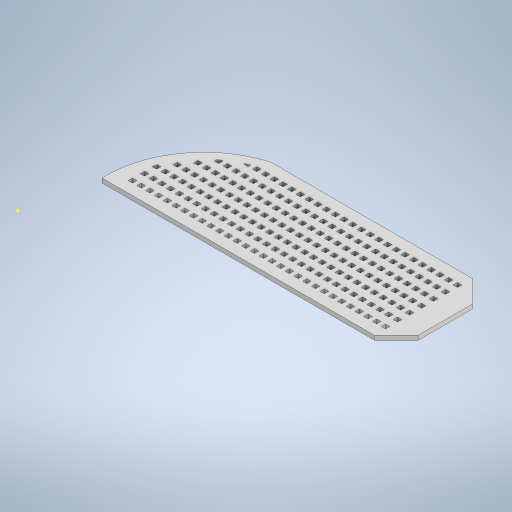
# Autodesk Inventor part: Cover_1
Saved by Autodesk Inventor 2024 (Build 280153000, 153)
## iProperties
Created: 2023-11-10
Part Number: Cover_1
Material: Generic
Document SubType Name: Modeling
Designer: furqa
Density: 1 g/cm^3
Appearance: Default
Author: furqa
Autodesk Inventor part; units mm, degrees
(part 1 of 2)
ref_plane "YZ Plane" through (0, 0, 0) normal (1, 0, 0) x (0, 1, 0)
ref_plane "XZ Plane" through (0, 0, 0) normal (0, 1, 0) x (-1, 0, 0)
ref_plane "XY Plane" through (0, 0, 0) normal (0, 0, 1) x (1, 0, 0)
sketch "Sketch1" plane through (0, 0, 0) normal (0, 1, 0) x (-1, 0, 0)
  line L0 (-38.923, -75.3658) -> (-131.4067, -75.3658)
  line L1 (-131.4067, -34.3658) -> (-8.4067, -34.3658)
  line L2 (-8.4067, -34.3658) -> (-8.4067, -37.0555)
  line L3 (-6.4067, -77.3658) -> (-6.4067, -32.3658)
  line L4 (-6.4067, -32.3658) -> (-131.4067, -32.3658)
  line L5 (-131.4067, -77.3658) -> (-6.4067, -77.3658)
  line L6 (-141.4067, -42.3658) -> (-141.4067, -67.3658)
  arc A0 (-38.923, -77.3658) -> (-6.4067, -33.3658) centre (-51.1866, -34.288) ccw
  arc A1 (-38.923, -75.3658) -> (-8.4067, -37.0555) centre (-51.1866, -34.288) ccw
  arc A2 (-131.4067, -34.3658) -> (-131.4067, -75.3658) centre (-62.8651, -54.8658) ccw
  line L7 (-131.4067, -77.3658) -> (-131.4067, -75.3658)
  line L8 (-131.4067, -34.3658) -> (-131.4067, -32.3658)
  line L9 (-189.1996, -35.8658) -> (-191.1996, -35.8658)
  line L10 (-191.1996, -35.8658) -> (-191.1996, -37.8658)
  line L11 (-191.1996, -37.8658) -> (-189.1996, -37.8658)
  line L12 (-189.1996, -37.8658) -> (-189.1996, -35.8658)
  line L13 (-6.4067, -32.3658) -> (-131.4067, -32.3658)
  line L14 (-131.4067, -32.3658) -> (-141.4067, -42.3658)
  line L15 (-141.4067, -42.3658) -> (-141.4067, -67.3658)
  line L16 (-141.4067, -67.3658) -> (-131.4067, -77.3658)
  line L17 (-131.4067, -77.3658) -> (-38.923, -77.3658)
  arc A3 (-38.923, -77.3658) -> (-6.4067, -32.3658) centre (-51.3198, -34.1601) ccw
  point P0 (-141.4067, -54.8658)
  point P1 (-131.4067, -54.8658)
  point P2 (-6.4067, -35.2102)
  point P3 (-131.4067, -54.8658)
  point P4 (-134.4067, -54.8658)
  point P5 (-7.6435, -44.7803)
  point P6 (-6.4067, -35.2102)
  dimension "d2" = 2
  dimension "d3" = 2
  dimension "d4" = 2
  dimension "d5" = 2
  dimension "d6" = 2
  dimension "d7" = 1.5
  constraints: 36 end point, 9 point on circle, 5 parallel, 4 centre point, 2 horizontal, 2 point on line, 2 vertical, 1 coincident, 1 collinear, 1 midpoint, 1 perpendicular
  measures "d2" distance between parallel lines of L3 L2
  measures "d3" distance between parallel lines of L4 L1
  measures "d4" distance between parallel lines of L5 L0
  measures "d5" distance of L9.start L9.end
  measures "d6" distance of L11.end L9.start
  measures "d7" distance between parallel lines of L1 L9
extrude "Extrusion1" add sketch "Sketch1" along normal blind 2 contours A1 L2 L1 L8 L4 L3 A0 A3 L5 L7 L0 | L0 A2 L1 L2 A1 | L7 L16 L6 L14 L8 A2 | A3 A0 | A0 L3 A3 picked at (-6.4675, -36.5311)
sketch "Sketch2" plane through (0, 0, 0) normal (0, -1, 0) x (1, 0, 0)
  circle A0 centre (8.4067, -35.3658) radius 0.95
  line L0 (6.4067, -32.3658) -> (131.4067, -32.3658) projected
  line L1 (6.4067, -35.2102) -> (6.4067, -32.3658) projected
  circle A1 centre (138.4067, -64.3658) radius 0.95
  circle A2 centre (138.4067, -45.3658) radius 0.95
  line L2 (131.4067, -77.3658) -> (38.923, -77.3658) projected
  line L3 (141.4067, -42.3658) -> (141.4067, -67.3658) projected
  point P0 (0, 0)
  dimension "d10" = 1.9
  dimension "d11" = 3
  dimension "d12" = 2
  dimension "d13" = 1.9
  dimension "d14" = 1.9
  dimension "d15" = 13
  dimension "d16" = 13
  dimension "d17" = 3
  dimension "d18" = 3
  constraints: 3 centre point
  measures "d10" diameter of A0
  measures "d11" distance from line of L0 A0.centre
  measures "d12" distance from line of L1 A0.centre
  measures "d13" diameter of A1
  measures "d14" diameter of A2
  measures "d15" distance from line of L2 A1.centre
  measures "d16" distance from line of L0 A2.centre
  measures "d17" distance from line of L3 A1.centre
  measures "d18" distance from line of L3 A2.centre
extrude "Extrusion2" add sketch "Sketch2" along normal blind 2
sketch "Sketch5" plane through (0, 2, 0) normal (0, 1, 0) x (1, 0, 0)
  point P0 (0, 0)
sketch "Sketch8" plane through (0, 2, 0) normal (0, 1, 0) x (1, 0, 0)
  point P0 (0, 0)
sketch "Sketch11" plane through (0, 2, 0) normal (0, 1, 0) x (1, 0, 0)
  line L0 (35.4067, 37.3658) -> (33.4067, 37.3658)
  line L1 (33.4067, 37.3658) -> (33.4067, 39.3658)
  line L2 (33.4067, 39.3658) -> (35.4067, 39.3658)
  line L3 (35.4067, 39.3658) -> (35.4067, 37.3658)
  line L4 (39.4067, 37.3658) -> (37.4067, 37.3658) projected
  line L5 (37.4067, 37.3658) -> (37.4067, 39.3658) projected
  line L6 (31.4067, 37.3658) -> (29.4067, 37.3658)
  line L7 (29.4067, 37.3658) -> (29.4067, 39.3658)
  line L8 (29.4067, 39.3658) -> (31.4067, 39.3658)
  line L9 (31.4067, 39.3658) -> (31.4067, 37.3658)
  line L10 (27.4067, 37.3658) -> (25.4067, 37.3658)
  line L11 (25.4067, 37.3658) -> (25.4067, 39.3658)
  line L12 (25.4067, 39.3658) -> (27.4067, 39.3658)
  line L13 (27.4067, 39.3658) -> (27.4067, 37.3658)
  line L14 (23.4067, 37.3658) -> (21.4067, 37.3658)
  line L15 (21.4067, 37.3658) -> (21.4067, 39.3658)
  line L16 (21.4067, 39.3658) -> (23.4067, 39.3658)
  line L17 (23.4067, 39.3658) -> (23.4067, 37.3658)
  line L18 (19.4067, 37.3658) -> (17.4067, 37.3658)
  line L19 (17.4067, 37.3658) -> (17.4067, 39.3658)
  line L20 (17.4067, 39.3658) -> (19.4067, 39.3658)
  line L21 (19.4067, 39.3658) -> (19.4067, 37.3658)
  line L22 (15.4067, 37.3658) -> (13.4067, 37.3658)
  line L23 (13.4067, 37.3658) -> (13.4067, 39.3658)
  line L24 (13.4067, 39.3658) -> (15.4067, 39.3658)
  line L25 (15.4067, 39.3658) -> (15.4067, 37.3658)
  line L26 (11.4067, 37.3658) -> (9.4067, 37.3658)
  line L27 (9.4067, 37.3658) -> (9.4067, 39.3658)
  line L28 (9.4067, 39.3658) -> (11.4067, 39.3658)
  line L29 (11.4067, 39.3658) -> (11.4067, 37.3658)
  line L30 (7.4067, 37.3658) -> (5.4067, 37.3658)
  line L31 (5.4067, 37.3658) -> (5.4067, 39.3658)
  line L32 (5.4067, 39.3658) -> (7.4067, 39.3658)
  line L33 (7.4067, 39.3658) -> (7.4067, 37.3658)
  line L34 (3.4067, 37.3658) -> (1.4067, 37.3658)
  line L35 (1.4067, 37.3658) -> (1.4067, 39.3658)
  line L36 (1.4067, 39.3658) -> (3.4067, 39.3658)
  line L37 (3.4067, 39.3658) -> (3.4067, 37.3658)
  line L38 (-0.5933, 37.3658) -> (-2.5933, 37.3658)
  line L39 (-2.5933, 37.3658) -> (-2.5933, 39.3658)
  line L40 (-2.5933, 39.3658) -> (-0.5933, 39.3658)
  line L41 (-0.5933, 39.3658) -> (-0.5933, 37.3658)
  line L42 (-4.5933, 37.3658) -> (-6.5933, 37.3658)
  line L43 (-6.5933, 37.3658) -> (-6.5933, 39.3658)
  line L44 (-6.5933, 39.3658) -> (-4.5933, 39.3658)
  line L45 (-4.5933, 39.3658) -> (-4.5933, 37.3658)
  line L46 (-8.5933, 37.3658) -> (-10.5933, 37.3658)
  line L47 (-10.5933, 37.3658) -> (-10.5933, 39.3658)
  line L48 (-10.5933, 39.3658) -> (-8.5933, 39.3658)
  line L49 (-8.5933, 39.3658) -> (-8.5933, 37.3658)
  line L50 (-12.5933, 37.3658) -> (-14.5933, 37.3658)
  line L51 (-14.5933, 37.3658) -> (-14.5933, 39.3658)
  line L52 (-14.5933, 39.3658) -> (-12.5933, 39.3658)
  line L53 (-12.5933, 39.3658) -> (-12.5933, 37.3658)
  line L54 (-16.5933, 37.3658) -> (-18.5933, 37.3658)
  line L55 (-18.5933, 37.3658) -> (-18.5933, 39.3658)
  line L56 (-18.5933, 39.3658) -> (-16.5933, 39.3658)
  line L57 (-16.5933, 39.3658) -> (-16.5933, 37.3658)
  line L58 (-20.5933, 37.3658) -> (-22.5933, 37.3658)
  line L59 (-22.5933, 37.3658) -> (-22.5933, 39.3658)
  line L60 (-22.5933, 39.3658) -> (-20.5933, 39.3658)
  line L61 (-20.5933, 39.3658) -> (-20.5933, 37.3658)
  line L62 (35.4067, 42.8658) -> (33.4067, 42.8658)
  line L63 (33.4067, 42.8658) -> (33.4067, 44.8658)
  line L64 (33.4067, 44.8658) -> (35.4067, 44.8658)
  line L65 (35.4067, 44.8658) -> (35.4067, 42.8658)
  line L66 (31.4067, 42.8658) -> (29.4067, 42.8658)
  line L67 (29.4067, 42.8658) -> (29.4067, 44.8658)
  line L68 (29.4067, 44.8658) -> (31.4067, 44.8658)
  line L69 (31.4067, 44.8658) -> (31.4067, 42.8658)
  line L70 (27.4067, 42.8658) -> (25.4067, 42.8658)
  line L71 (25.4067, 42.8658) -> (25.4067, 44.8658)
  line L72 (25.4067, 44.8658) -> (27.4067, 44.8658)
  line L73 (27.4067, 44.8658) -> (27.4067, 42.8658)
  line L74 (23.4067, 42.8658) -> (21.4067, 42.8658)
  line L75 (21.4067, 42.8658) -> (21.4067, 44.8658)
  line L76 (21.4067, 44.8658) -> (23.4067, 44.8658)
  line L77 (23.4067, 44.8658) -> (23.4067, 42.8658)
  line L78 (19.4067, 42.8658) -> (17.4067, 42.8658)
  line L79 (17.4067, 42.8658) -> (17.4067, 44.8658)
  line L80 (17.4067, 44.8658) -> (19.4067, 44.8658)
  line L81 (19.4067, 44.8658) -> (19.4067, 42.8658)
  line L82 (15.4067, 42.8658) -> (13.4067, 42.8658)
  line L83 (13.4067, 42.8658) -> (13.4067, 44.8658)
  line L84 (13.4067, 44.8658) -> (15.4067, 44.8658)
  line L85 (15.4067, 44.8658) -> (15.4067, 42.8658)
  line L86 (11.4067, 42.8658) -> (9.4067, 42.8658)
  line L87 (9.4067, 42.8658) -> (9.4067, 44.8658)
  line L88 (9.4067, 44.8658) -> (11.4067, 44.8658)
  line L89 (11.4067, 44.8658) -> (11.4067, 42.8658)
  line L90 (7.4067, 42.8658) -> (5.4067, 42.8658)
  line L91 (5.4067, 42.8658) -> (5.4067, 44.8658)
  line L92 (5.4067, 44.8658) -> (7.4067, 44.8658)
  line L93 (7.4067, 44.8658) -> (7.4067, 42.8658)
  line L94 (3.4067, 42.8658) -> (1.4067, 42.8658)
  line L95 (1.4067, 42.8658) -> (1.4067, 44.8658)
  line L96 (1.4067, 44.8658) -> (3.4067, 44.8658)
  line L97 (3.4067, 44.8658) -> (3.4067, 42.8658)
  line L98 (-0.5933, 42.8658) -> (-2.5933, 42.8658)
  line L99 (-2.5933, 42.8658) -> (-2.5933, 44.8658)
  line L100 (-2.5933, 44.8658) -> (-0.5933, 44.8658)
  line L101 (-0.5933, 44.8658) -> (-0.5933, 42.8658)
  line L102 (-4.5933, 42.8658) -> (-6.5933, 42.8658)
  line L103 (-6.5933, 42.8658) -> (-6.5933, 44.8658)
  line L104 (-6.5933, 44.8658) -> (-4.5933, 44.8658)
  line L105 (-4.5933, 44.8658) -> (-4.5933, 42.8658)
  line L106 (-8.5933, 42.8658) -> (-10.5933, 42.8658)
  line L107 (-10.5933, 42.8658) -> (-10.5933, 44.8658)
  line L108 (-10.5933, 44.8658) -> (-8.5933, 44.8658)
  line L109 (-8.5933, 44.8658) -> (-8.5933, 42.8658)
  line L110 (-12.5933, 42.8658) -> (-14.5933, 42.8658)
  line L111 (-14.5933, 42.8658) -> (-14.5933, 44.8658)
  line L112 (-14.5933, 44.8658) -> (-12.5933, 44.8658)
  line L113 (-12.5933, 44.8658) -> (-12.5933, 42.8658)
  line L114 (-16.5933, 42.8658) -> (-18.5933, 42.8658)
  line L115 (-18.5933, 42.8658) -> (-18.5933, 44.8658)
  line L116 (-18.5933, 44.8658) -> (-16.5933, 44.8658)
  line L117 (-16.5933, 44.8658) -> (-16.5933, 42.8658)
  line L118 (-20.5933, 42.8658) -> (-22.5933, 42.8658)
  line L119 (-22.5933, 42.8658) -> (-22.5933, 44.8658)
  line L120 (-22.5933, 44.8658) -> (-20.5933, 44.8658)
  line L121 (-20.5933, 44.8658) -> (-20.5933, 42.8658)
  line L122 (35.4067, 48.3658) -> (33.4067, 48.3658)
  line L123 (33.4067, 48.3658) -> (33.4067, 50.3658)
  line L124 (33.4067, 50.3658) -> (35.4067, 50.3658)
  line L125 (35.4067, 50.3658) -> (35.4067, 48.3658)
  line L126 (31.4067, 48.3658) -> (29.4067, 48.3658)
  line L127 (29.4067, 48.3658) -> (29.4067, 50.3658)
  line L128 (29.4067, 50.3658) -> (31.4067, 50.3658)
  line L129 (31.4067, 50.3658) -> (31.4067, 48.3658)
  line L130 (27.4067, 48.3658) -> (25.4067, 48.3658)
  line L131 (25.4067, 48.3658) -> (25.4067, 50.3658)
  line L132 (25.4067, 50.3658) -> (27.4067, 50.3658)
  line L133 (27.4067, 50.3658) -> (27.4067, 48.3658)
  line L134 (23.4067, 48.3658) -> (21.4067, 48.3658)
  line L135 (21.4067, 48.3658) -> (21.4067, 50.3658)
  line L136 (21.4067, 50.3658) -> (23.4067, 50.3658)
  line L137 (23.4067, 50.3658) -> (23.4067, 48.3658)
  line L138 (19.4067, 48.3658) -> (17.4067, 48.3658)
  line L139 (17.4067, 48.3658) -> (17.4067, 50.3658)
  line L140 (17.4067, 50.3658) -> (19.4067, 50.3658)
  line L141 (19.4067, 50.3658) -> (19.4067, 48.3658)
  line L142 (15.4067, 48.3658) -> (13.4067, 48.3658)
  line L143 (13.4067, 48.3658) -> (13.4067, 50.3658)
  line L144 (13.4067, 50.3658) -> (15.4067, 50.3658)
  line L145 (15.4067, 50.3658) -> (15.4067, 48.3658)
  line L146 (11.4067, 48.3658) -> (9.4067, 48.3658)
  line L147 (9.4067, 48.3658) -> (9.4067, 50.3658)
  line L148 (9.4067, 50.3658) -> (11.4067, 50.3658)
  line L149 (11.4067, 50.3658) -> (11.4067, 48.3658)
  line L150 (7.4067, 48.3658) -> (5.4067, 48.3658)
  line L151 (5.4067, 48.3658) -> (5.4067, 50.3658)
  line L152 (5.4067, 50.3658) -> (7.4067, 50.3658)
  line L153 (7.4067, 50.3658) -> (7.4067, 48.3658)
  line L154 (3.4067, 48.3658) -> (1.4067, 48.3658)
  line L155 (1.4067, 48.3658) -> (1.4067, 50.3658)
  line L156 (1.4067, 50.3658) -> (3.4067, 50.3658)
  line L157 (3.4067, 50.3658) -> (3.4067, 48.3658)
  line L158 (-0.5933, 48.3658) -> (-2.5933, 48.3658)
  line L159 (-2.5933, 48.3658) -> (-2.5933, 50.3658)
  line L160 (-2.5933, 50.3658) -> (-0.5933, 50.3658)
  line L161 (-0.5933, 50.3658) -> (-0.5933, 48.3658)
  line L162 (-4.5933, 48.3658) -> (-6.5933, 48.3658)
  line L163 (-6.5933, 48.3658) -> (-6.5933, 50.3658)
  line L164 (-6.5933, 50.3658) -> (-4.5933, 50.3658)
  line L165 (-4.5933, 50.3658) -> (-4.5933, 48.3658)
  line L166 (-8.5933, 48.3658) -> (-10.5933, 48.3658)
  line L167 (-10.5933, 48.3658) -> (-10.5933, 50.3658)
  line L168 (-10.5933, 50.3658) -> (-8.5933, 50.3658)
  line L169 (-8.5933, 50.3658) -> (-8.5933, 48.3658)
  line L170 (-12.5933, 48.3658) -> (-14.5933, 48.3658)
  line L171 (-14.5933, 48.3658) -> (-14.5933, 50.3658)
  line L172 (-14.5933, 50.3658) -> (-12.5933, 50.3658)
  line L173 (-12.5933, 50.3658) -> (-12.5933, 48.3658)
  line L174 (-16.5933, 48.3658) -> (-18.5933, 48.3658)
  line L175 (-18.5933, 48.3658) -> (-18.5933, 50.3658)
  line L176 (-18.5933, 50.3658) -> (-16.5933, 50.3658)
  line L177 (-16.5933, 50.3658) -> (-16.5933, 48.3658)
  line L178 (-20.5933, 48.3658) -> (-22.5933, 48.3658)
  line L179 (-22.5933, 48.3658) -> (-22.5933, 50.3658)
  line L180 (-22.5933, 50.3658) -> (-20.5933, 50.3658)
  line L181 (-20.5933, 50.3658) -> (-20.5933, 48.3658)
  line L182 (35.4067, 53.8658) -> (33.4067, 53.8658)
  line L183 (33.4067, 53.8658) -> (33.4067, 55.8658)
  line L184 (33.4067, 55.8658) -> (35.4067, 55.8658)
  line L185 (35.4067, 55.8658) -> (35.4067, 53.8658)
  line L186 (31.4067, 53.8658) -> (29.4067, 53.8658)
  line L187 (29.4067, 53.8658) -> (29.4067, 55.8658)
  line L188 (29.4067, 55.8658) -> (31.4067, 55.8658)
  line L189 (31.4067, 55.8658) -> (31.4067, 53.8658)
  line L190 (27.4067, 53.8658) -> (25.4067, 53.8658)
  line L191 (25.4067, 53.8658) -> (25.4067, 55.8658)
  line L192 (25.4067, 55.8658) -> (27.4067, 55.8658)
  line L193 (27.4067, 55.8658) -> (27.4067, 53.8658)
  line L194 (23.4067, 53.8658) -> (21.4067, 53.8658)
  line L195 (21.4067, 53.8658) -> (21.4067, 55.8658)
  line L196 (21.4067, 55.8658) -> (23.4067, 55.8658)
  line L197 (23.4067, 55.8658) -> (23.4067, 53.8658)
  line L198 (19.4067, 53.8658) -> (17.4067, 53.8658)
  line L199 (17.4067, 53.8658) -> (17.4067, 55.8658)
  line L200 (17.4067, 55.8658) -> (19.4067, 55.8658)
  line L201 (19.4067, 55.8658) -> (19.4067, 53.8658)
  line L202 (15.4067, 53.8658) -> (13.4067, 53.8658)
  line L203 (13.4067, 53.8658) -> (13.4067, 55.8658)
  line L204 (13.4067, 55.8658) -> (15.4067, 55.8658)
  line L205 (15.4067, 55.8658) -> (15.4067, 53.8658)
  line L206 (11.4067, 53.8658) -> (9.4067, 53.8658)
  line L207 (9.4067, 53.8658) -> (9.4067, 55.8658)
  line L208 (9.4067, 55.8658) -> (11.4067, 55.8658)
  line L209 (11.4067, 55.8658) -> (11.4067, 53.8658)
  line L210 (7.4067, 53.8658) -> (5.4067, 53.8658)
  line L211 (5.4067, 53.8658) -> (5.4067, 55.8658)
  line L212 (5.4067, 55.8658) -> (7.4067, 55.8658)
  line L213 (7.4067, 55.8658) -> (7.4067, 53.8658)
  line L214 (3.4067, 53.8658) -> (1.4067, 53.8658)
  line L215 (1.4067, 53.8658) -> (1.4067, 55.8658)
  line L216 (1.4067, 55.8658) -> (3.4067, 55.8658)
  line L217 (3.4067, 55.8658) -> (3.4067, 53.8658)
  line L218 (-0.5933, 53.8658) -> (-2.5933, 53.8658)
  line L219 (-2.5933, 53.8658) -> (-2.5933, 55.8658)
  line L220 (-2.5933, 55.8658) -> (-0.5933, 55.8658)
  line L221 (-0.5933, 55.8658) -> (-0.5933, 53.8658)
  line L222 (-4.5933, 53.8658) -> (-6.5933, 53.8658)
  line L223 (-6.5933, 53.8658) -> (-6.5933, 55.8658)
  line L224 (-6.5933, 55.8658) -> (-4.5933, 55.8658)
  line L225 (-4.5933, 55.8658) -> (-4.5933, 53.8658)
  line L226 (-8.5933, 53.8658) -> (-10.5933, 53.8658)
  line L227 (-10.5933, 53.8658) -> (-10.5933, 55.8658)
  line L228 (-10.5933, 55.8658) -> (-8.5933, 55.8658)
  line L229 (-8.5933, 55.8658) -> (-8.5933, 53.8658)
  line L230 (-12.5933, 53.8658) -> (-14.5933, 53.8658)
  line L231 (-14.5933, 53.8658) -> (-14.5933, 55.8658)
  line L232 (-14.5933, 55.8658) -> (-12.5933, 55.8658)
  line L233 (-12.5933, 55.8658) -> (-12.5933, 53.8658)
  line L234 (-16.5933, 53.8658) -> (-18.5933, 53.8658)
  line L235 (-18.5933, 53.8658) -> (-18.5933, 55.8658)
  line L236 (-18.5933, 55.8658) -> (-16.5933, 55.8658)
  line L237 (-16.5933, 55.8658) -> (-16.5933, 53.8658)
  line L238 (-20.5933, 53.8658) -> (-22.5933, 53.8658)
  line L239 (-22.5933, 53.8658) -> (-22.5933, 55.8658)
  line L240 (-22.5933, 55.8658) -> (-20.5933, 55.8658)
  line L241 (-20.5933, 55.8658) -> (-20.5933, 53.8658)
  line L242 (35.4067, 59.3658) -> (33.4067, 59.3658)
  line L243 (33.4067, 59.3658) -> (33.4067, 61.3658)
  line L244 (33.4067, 61.3658) -> (35.4067, 61.3658)
  line L245 (35.4067, 61.3658) -> (35.4067, 59.3658)
  line L246 (31.4067, 59.3658) -> (29.4067, 59.3658)
  line L247 (29.4067, 59.3658) -> (29.4067, 61.3658)
  line L248 (29.4067, 61.3658) -> (31.4067, 61.3658)
  line L249 (31.4067, 61.3658) -> (31.4067, 59.3658)
  line L250 (27.4067, 59.3658) -> (25.4067, 59.3658)
  line L251 (25.4067, 59.3658) -> (25.4067, 61.3658)
  line L252 (25.4067, 61.3658) -> (27.4067, 61.3658)
  line L253 (27.4067, 61.3658) -> (27.4067, 59.3658)
  line L254 (23.4067, 59.3658) -> (21.4067, 59.3658)
  line L255 (21.4067, 59.3658) -> (21.4067, 61.3658)
  line L256 (21.4067, 61.3658) -> (23.4067, 61.3658)
  line L257 (23.4067, 61.3658) -> (23.4067, 59.3658)
  line L258 (19.4067, 59.3658) -> (17.4067, 59.3658)
  line L259 (17.4067, 59.3658) -> (17.4067, 61.3658)
  line L260 (17.4067, 61.3658) -> (19.4067, 61.3658)
  line L261 (19.4067, 61.3658) -> (19.4067, 59.3658)
  line L262 (15.4067, 59.3658) -> (13.4067, 59.3658)
  line L263 (13.4067, 59.3658) -> (13.4067, 61.3658)
  line L264 (13.4067, 61.3658) -> (15.4067, 61.3658)
  line L265 (15.4067, 61.3658) -> (15.4067, 59.3658)
  line L266 (11.4067, 59.3658) -> (9.4067, 59.3658)
  line L267 (9.4067, 59.3658) -> (9.4067, 61.3658)
  line L268 (9.4067, 61.3658) -> (11.4067, 61.3658)
  line L269 (11.4067, 61.3658) -> (11.4067, 59.3658)
  line L270 (7.4067, 59.3658) -> (5.4067, 59.3658)
  line L271 (5.4067, 59.3658) -> (5.4067, 61.3658)
  line L272 (5.4067, 61.3658) -> (7.4067, 61.3658)
  line L273 (7.4067, 61.3658) -> (7.4067, 59.3658)
  line L274 (3.4067, 59.3658) -> (1.4067, 59.3658)
  line L275 (1.4067, 59.3658) -> (1.4067, 61.3658)
  line L276 (1.4067, 61.3658) -> (3.4067, 61.3658)
  line L277 (3.4067, 61.3658) -> (3.4067, 59.3658)
  line L278 (-0.5933, 59.3658) -> (-2.5933, 59.3658)
  line L279 (-2.5933, 59.3658) -> (-2.5933, 61.3658)
  line L280 (-2.5933, 61.3658) -> (-0.5933, 61.3658)
  line L281 (-0.5933, 61.3658) -> (-0.5933, 59.3658)
  line L282 (-4.5933, 59.3658) -> (-6.5933, 59.3658)
  line L283 (-6.5933, 59.3658) -> (-6.5933, 61.3658)
  line L284 (-6.5933, 61.3658) -> (-4.5933, 61.3658)
  line L285 (-4.5933, 61.3658) -> (-4.5933, 59.3658)
  line L286 (-8.5933, 59.3658) -> (-10.5933, 59.3658)
  line L287 (-10.5933, 59.3658) -> (-10.5933, 61.3658)
  line L288 (-10.5933, 61.3658) -> (-8.5933, 61.3658)
  line L289 (-8.5933, 61.3658) -> (-8.5933, 59.3658)
  line L290 (-12.5933, 59.3658) -> (-14.5933, 59.3658)
  line L291 (-14.5933, 59.3658) -> (-14.5933, 61.3658)
  line L292 (-14.5933, 61.3658) -> (-12.5933, 61.3658)
  line L293 (-12.5933, 61.3658) -> (-12.5933, 59.3658)
  line L294 (-16.5933, 59.3658) -> (-18.5933, 59.3658)
  line L295 (-18.5933, 59.3658) -> (-18.5933, 61.3658)
  line L296 (-18.5933, 61.3658) -> (-16.5933, 61.3658)
  line L297 (-16.5933, 61.3658) -> (-16.5933, 59.3658)
  line L298 (-20.5933, 59.3658) -> (-22.5933, 59.3658)
  line L299 (-22.5933, 59.3658) -> (-22.5933, 61.3658)
  line L300 (-22.5933, 61.3658) -> (-20.5933, 61.3658)
  line L301 (-20.5933, 61.3658) -> (-20.5933, 59.3658)
  line L302 (35.4067, 64.8658) -> (33.4067, 64.8658)
  line L303 (33.4067, 64.8658) -> (33.4067, 66.8658)
  line L304 (33.4067, 66.8658) -> (35.4067, 66.8658)
  line L305 (35.4067, 66.8658) -> (35.4067, 64.8658)
  line L306 (31.4067, 64.8658) -> (29.4067, 64.8658)
  line L307 (29.4067, 64.8658) -> (29.4067, 66.8658)
  line L308 (29.4067, 66.8658) -> (31.4067, 66.8658)
  line L309 (31.4067, 66.8658) -> (31.4067, 64.8658)
  line L310 (27.4067, 64.8658) -> (25.4067, 64.8658)
  line L311 (25.4067, 64.8658) -> (25.4067, 66.8658)
  line L312 (25.4067, 66.8658) -> (27.4067, 66.8658)
  line L313 (27.4067, 66.8658) -> (27.4067, 64.8658)
  line L314 (23.4067, 64.8658) -> (21.4067, 64.8658)
  line L315 (21.4067, 64.8658) -> (21.4067, 66.8658)
  line L316 (21.4067, 66.8658) -> (23.4067, 66.8658)
  line L317 (23.4067, 66.8658) -> (23.4067, 64.8658)
  line L318 (19.4067, 64.8658) -> (17.4067, 64.8658)
  line L319 (17.4067, 64.8658) -> (17.4067, 66.8658)
  line L320 (17.4067, 66.8658) -> (19.4067, 66.8658)
  line L321 (19.4067, 66.8658) -> (19.4067, 64.8658)
  line L322 (15.4067, 64.8658) -> (13.4067, 64.8658)
  line L323 (13.4067, 64.8658) -> (13.4067, 66.8658)
  line L324 (13.4067, 66.8658) -> (15.4067, 66.8658)
  line L325 (15.4067, 66.8658) -> (15.4067, 64.8658)
  line L326 (11.4067, 64.8658) -> (9.4067, 64.8658)
  line L327 (9.4067, 64.8658) -> (9.4067, 66.8658)
  line L328 (9.4067, 66.8658) -> (11.4067, 66.8658)
  line L329 (11.4067, 66.8658) -> (11.4067, 64.8658)
  line L330 (7.4067, 64.8658) -> (5.4067, 64.8658)
  line L331 (5.4067, 64.8658) -> (5.4067, 66.8658)
  line L332 (5.4067, 66.8658) -> (7.4067, 66.8658)
  line L333 (7.4067, 66.8658) -> (7.4067, 64.8658)
  line L334 (3.4067, 64.8658) -> (1.4067, 64.8658)
  line L335 (1.4067, 64.8658) -> (1.4067, 66.8658)
  line L336 (1.4067, 66.8658) -> (3.4067, 66.8658)
  line L337 (3.4067, 66.8658) -> (3.4067, 64.8658)
  line L338 (-0.5933, 64.8658) -> (-2.5933, 64.8658)
  line L339 (-2.5933, 64.8658) -> (-2.5933, 66.8658)
  line L340 (-2.5933, 66.8658) -> (-0.5933, 66.8658)
  line L341 (-0.5933, 66.8658) -> (-0.5933, 64.8658)
  line L342 (-4.5933, 64.8658) -> (-6.5933, 64.8658)
  line L343 (-6.5933, 64.8658) -> (-6.5933, 66.8658)
  line L344 (-6.5933, 66.8658) -> (-4.5933, 66.8658)
  line L345 (-4.5933, 66.8658) -> (-4.5933, 64.8658)
  line L346 (-8.5933, 64.8658) -> (-10.5933, 64.8658)
  line L347 (-10.5933, 64.8658) -> (-10.5933, 66.8658)
  line L348 (-10.5933, 66.8658) -> (-8.5933, 66.8658)
  line L349 (-8.5933, 66.8658) -> (-8.5933, 64.8658)
  line L350 (-12.5933, 64.8658) -> (-14.5933, 64.8658)
  line L351 (-14.5933, 64.8658) -> (-14.5933, 66.8658)
  line L352 (-14.5933, 66.8658) -> (-12.5933, 66.8658)
  line L353 (-12.5933, 66.8658) -> (-12.5933, 64.8658)
  line L354 (-16.5933, 64.8658) -> (-18.5933, 64.8658)
  line L355 (-18.5933, 64.8658) -> (-18.5933, 66.8658)
  line L356 (-18.5933, 66.8658) -> (-16.5933, 66.8658)
  line L357 (-16.5933, 66.8658) -> (-16.5933, 64.8658)
  line L358 (-20.5933, 64.8658) -> (-22.5933, 64.8658)
  line L359 (-22.5933, 64.8658) -> (-22.5933, 66.8658)
  line L360 (-22.5933, 66.8658) -> (-20.5933, 66.8658)
  line L361 (-20.5933, 66.8658) -> (-20.5933, 64.8658)
  line L362 (35.4067, 70.3658) -> (33.4067, 70.3658)
  line L363 (33.4067, 70.3658) -> (33.4067, 72.3658)
  line L364 (33.4067, 72.3658) -> (35.4067, 72.3658)
  line L365 (35.4067, 72.3658) -> (35.4067, 70.3658)
  line L366 (31.4067, 70.3658) -> (29.4067, 70.3658)
  line L367 (29.4067, 70.3658) -> (29.4067, 72.3658)
  line L368 (29.4067, 72.3658) -> (31.4067, 72.3658)
  line L369 (31.4067, 72.3658) -> (31.4067, 70.3658)
  line L370 (27.4067, 70.3658) -> (25.4067, 70.3658)
  line L371 (25.4067, 70.3658) -> (25.4067, 72.3658)
  line L372 (25.4067, 72.3658) -> (27.4067, 72.3658)
  line L373 (27.4067, 72.3658) -> (27.4067, 70.3658)
  line L374 (23.4067, 70.3658) -> (21.4067, 70.3658)
  line L375 (21.4067, 70.3658) -> (21.4067, 72.3658)
  line L376 (21.4067, 72.3658) -> (23.4067, 72.3658)
  line L377 (23.4067, 72.3658) -> (23.4067, 70.3658)
  line L378 (19.4067, 70.3658) -> (17.4067, 70.3658)
  line L379 (17.4067, 70.3658) -> (17.4067, 72.3658)
  line L380 (17.4067, 72.3658) -> (19.4067, 72.3658)
  line L381 (19.4067, 72.3658) -> (19.4067, 70.3658)
  line L382 (15.4067, 70.3658) -> (13.4067, 70.3658)
  line L383 (13.4067, 70.3658) -> (13.4067, 72.3658)
  line L384 (13.4067, 72.3658) -> (15.4067, 72.3658)
  line L385 (15.4067, 72.3658) -> (15.4067, 70.3658)
  line L386 (11.4067, 70.3658) -> (9.4067, 70.3658)
  line L387 (9.4067, 70.3658) -> (9.4067, 72.3658)
  line L388 (9.4067, 72.3658) -> (11.4067, 72.3658)
  line L389 (11.4067, 72.3658) -> (11.4067, 70.3658)
  line L390 (7.4067, 70.3658) -> (5.4067, 70.3658)
  line L391 (5.4067, 70.3658) -> (5.4067, 72.3658)
  line L392 (5.4067, 72.3658) -> (7.4067, 72.3658)
  line L393 (7.4067, 72.3658) -> (7.4067, 70.3658)
  line L394 (3.4067, 70.3658) -> (1.4067, 70.3658)
  line L395 (1.4067, 70.3658) -> (1.4067, 72.3658)
  line L396 (1.4067, 72.3658) -> (3.4067, 72.3658)
  line L397 (3.4067, 72.3658) -> (3.4067, 70.3658)
  line L398 (-0.5933, 70.3658) -> (-2.5933, 70.3658)
  line L399 (-2.5933, 70.3658) -> (-2.5933, 72.3658)
  line L400 (-2.5933, 72.3658) -> (-0.5933, 72.3658)
  line L401 (-0.5933, 72.3658) -> (-0.5933, 70.3658)
  line L402 (-4.5933, 70.3658) -> (-6.5933, 70.3658)
  line L403 (-6.5933, 70.3658) -> (-6.5933, 72.3658)
  line L404 (-6.5933, 72.3658) -> (-4.5933, 72.3658)
  line L405 (-4.5933, 72.3658) -> (-4.5933, 70.3658)
  line L406 (-8.5933, 70.3658) -> (-10.5933, 70.3658)
  line L407 (-10.5933, 70.3658) -> (-10.5933, 72.3658)
  line L408 (-10.5933, 72.3658) -> (-8.5933, 72.3658)
  line L409 (-8.5933, 72.3658) -> (-8.5933, 70.3658)
  line L410 (-12.5933, 70.3658) -> (-14.5933, 70.3658)
  line L411 (-14.5933, 70.3658) -> (-14.5933, 72.3658)
  line L412 (-14.5933, 72.3658) -> (-12.5933, 72.3658)
  line L413 (-12.5933, 72.3658) -> (-12.5933, 70.3658)
  line L414 (-16.5933, 70.3658) -> (-18.5933, 70.3658)
  line L415 (-18.5933, 70.3658) -> (-18.5933, 72.3658)
  line L416 (-18.5933, 72.3658) -> (-16.5933, 72.3658)
  line L417 (-16.5933, 72.3658) -> (-16.5933, 70.3658)
  line L418 (-20.5933, 70.3658) -> (-22.5933, 70.3658)
  line L419 (-22.5933, 70.3658) -> (-22.5933, 72.3658)
  line L420 (-22.5933, 72.3658) -> (-20.5933, 72.3658)
  line L421 (-20.5933, 72.3658) -> (-20.5933, 70.3658)
  line L422 (35.4067, 75.8658) -> (33.4067, 75.8658)
  line L423 (33.4067, 75.8658) -> (33.4067, 77.8658)
  line L424 (33.4067, 77.8658) -> (35.4067, 77.8658)
  line L425 (35.4067, 77.8658) -> (35.4067, 75.8658)
  line L426 (31.4067, 75.8658) -> (29.4067, 75.8658)
  line L427 (29.4067, 75.8658) -> (29.4067, 77.8658)
  line L428 (29.4067, 77.8658) -> (31.4067, 77.8658)
  line L429 (31.4067, 77.8658) -> (31.4067, 75.8658)
  line L430 (27.4067, 75.8658) -> (25.4067, 75.8658)
  line L431 (25.4067, 75.8658) -> (25.4067, 77.8658)
  line L432 (25.4067, 77.8658) -> (27.4067, 77.8658)
  line L433 (27.4067, 77.8658) -> (27.4067, 75.8658)
  line L434 (23.4067, 75.8658) -> (21.4067, 75.8658)
  line L435 (21.4067, 75.8658) -> (21.4067, 77.8658)
  line L436 (21.4067, 77.8658) -> (23.4067, 77.8658)
  line L437 (23.4067, 77.8658) -> (23.4067, 75.8658)
  line L438 (19.4067, 75.8658) -> (17.4067, 75.8658)
  line L439 (17.4067, 75.8658) -> (17.4067, 77.8658)
  line L440 (17.4067, 77.8658) -> (19.4067, 77.8658)
  line L441 (19.4067, 77.8658) -> (19.4067, 75.8658)
  line L442 (15.4067, 75.8658) -> (13.4067, 75.8658)
  line L443 (13.4067, 75.8658) -> (13.4067, 77.8658)
  line L444 (13.4067, 77.8658) -> (15.4067, 77.8658)
  line L445 (15.4067, 77.8658) -> (15.4067, 75.8658)
  line L446 (11.4067, 75.8658) -> (9.4067, 75.8658)
  line L447 (9.4067, 75.8658) -> (9.4067, 77.8658)
  line L448 (9.4067, 77.8658) -> (11.4067, 77.8658)
  line L449 (11.4067, 77.8658) -> (11.4067, 75.8658)
  line L450 (7.4067, 75.8658) -> (5.4067, 75.8658)
  line L451 (5.4067, 75.8658) -> (5.4067, 77.8658)
  line L452 (5.4067, 77.8658) -> (7.4067, 77.8658)
  line L453 (7.4067, 77.8658) -> (7.4067, 75.8658)
  line L454 (3.4067, 75.8658) -> (1.4067, 75.8658)
  line L455 (1.4067, 75.8658) -> (1.4067, 77.8658)
  line L456 (1.4067, 77.8658) -> (3.4067, 77.8658)
  line L457 (3.4067, 77.8658) -> (3.4067, 75.8658)
  line L458 (-0.5933, 75.8658) -> (-2.5933, 75.8658)
  line L459 (-2.5933, 75.8658) -> (-2.5933, 77.8658)
  line L460 (-2.5933, 77.8658) -> (-0.5933, 77.8658)
  line L461 (-0.5933, 77.8658) -> (-0.5933, 75.8658)
  line L462 (-4.5933, 75.8658) -> (-6.5933, 75.8658)
  line L463 (-6.5933, 75.8658) -> (-6.5933, 77.8658)
  line L464 (-6.5933, 77.8658) -> (-4.5933, 77.8658)
  line L465 (-4.5933, 77.8658) -> (-4.5933, 75.8658)
  line L466 (-8.5933, 75.8658) -> (-10.5933, 75.8658)
  line L467 (-10.5933, 75.8658) -> (-10.5933, 77.8658)
  line L468 (-10.5933, 77.8658) -> (-8.5933, 77.8658)
  line L469 (-8.5933, 77.8658) -> (-8.5933, 75.8658)
  line L470 (-12.5933, 75.8658) -> (-14.5933, 75.8658)
  line L471 (-14.5933, 75.8658) -> (-14.5933, 77.8658)
  line L472 (-14.5933, 77.8658) -> (-12.5933, 77.8658)
  line L473 (-12.5933, 77.8658) -> (-12.5933, 75.8658)
  line L474 (-16.5933, 75.8658) -> (-18.5933, 75.8658)
  line L475 (-18.5933, 75.8658) -> (-18.5933, 77.8658)
  line L476 (-18.5933, 77.8658) -> (-16.5933, 77.8658)
  line L477 (-16.5933, 77.8658) -> (-16.5933, 75.8658)
  line L478 (-20.5933, 75.8658) -> (-22.5933, 75.8658)
  line L479 (-22.5933, 75.8658) -> (-22.5933, 77.8658)
  line L480 (-22.5933, 77.8658) -> (-20.5933, 77.8658)
  line L481 (-20.5933, 77.8658) -> (-20.5933, 75.8658)
  line L482 (35.4067, 81.3658) -> (33.4067, 81.3658)
  line L483 (33.4067, 81.3658) -> (33.4067, 83.3658)
  line L484 (33.4067, 83.3658) -> (35.4067, 83.3658)
  line L485 (35.4067, 83.3658) -> (35.4067, 81.3658)
  line L486 (31.4067, 81.3658) -> (29.4067, 81.3658)
  line L487 (29.4067, 81.3658) -> (29.4067, 83.3658)
  line L488 (29.4067, 83.3658) -> (31.4067, 83.3658)
  line L489 (31.4067, 83.3658) -> (31.4067, 81.3658)
  line L490 (27.4067, 81.3658) -> (25.4067, 81.3658)
  line L491 (25.4067, 81.3658) -> (25.4067, 83.3658)
  line L492 (25.4067, 83.3658) -> (27.4067, 83.3658)
  line L493 (27.4067, 83.3658) -> (27.4067, 81.3658)
  line L494 (23.4067, 81.3658) -> (21.4067, 81.3658)
  line L495 (21.4067, 81.3658) -> (21.4067, 83.3658)
  line L496 (21.4067, 83.3658) -> (23.4067, 83.3658)
  line L497 (23.4067, 83.3658) -> (23.4067, 81.3658)
  line L498 (19.4067, 81.3658) -> (17.4067, 81.3658)
  line L499 (17.4067, 81.3658) -> (17.4067, 83.3658)
  line L500 (17.4067, 83.3658) -> (19.4067, 83.3658)
  line L501 (19.4067, 83.3658) -> (19.4067, 81.3658)
  line L502 (15.4067, 81.3658) -> (13.4067, 81.3658)
  line L503 (13.4067, 81.3658) -> (13.4067, 83.3658)
  line L504 (13.4067, 83.3658) -> (15.4067, 83.3658)
  line L505 (15.4067, 83.3658) -> (15.4067, 81.3658)
  line L506 (11.4067, 81.3658) -> (9.4067, 81.3658)
  line L507 (9.4067, 81.3658) -> (9.4067, 83.3658)
  line L508 (9.4067, 83.3658) -> (11.4067, 83.3658)
  line L509 (11.4067, 83.3658) -> (11.4067, 81.3658)
  line L510 (7.4067, 81.3658) -> (5.4067, 81.3658)
  line L511 (5.4067, 81.3658) -> (5.4067, 83.3658)
  line L512 (5.4067, 83.3658) -> (7.4067, 83.3658)
  line L513 (7.4067, 83.3658) -> (7.4067, 81.3658)
  line L514 (3.4067, 81.3658) -> (1.4067, 81.3658)
  line L515 (1.4067, 81.3658) -> (1.4067, 83.3658)
  line L516 (1.4067, 83.3658) -> (3.4067, 83.3658)
  line L517 (3.4067, 83.3658) -> (3.4067, 81.3658)
  line L518 (-0.5933, 81.3658) -> (-2.5933, 81.3658)
  line L519 (-2.5933, 81.3658) -> (-2.5933, 83.3658)
  line L520 (-2.5933, 83.3658) -> (-0.5933, 83.3658)
  line L521 (-0.5933, 83.3658) -> (-0.5933, 81.3658)
  line L522 (-4.5933, 81.3658) -> (-6.5933, 81.3658)
  line L523 (-6.5933, 81.3658) -> (-6.5933, 83.3658)
  line L524 (-6.5933, 83.3658) -> (-4.5933, 83.3658)
  line L525 (-4.5933, 83.3658) -> (-4.5933, 81.3658)
  line L526 (-8.5933, 81.3658) -> (-10.5933, 81.3658)
  line L527 (-10.5933, 81.3658) -> (-10.5933, 83.3658)
  line L528 (-10.5933, 83.3658) -> (-8.5933, 83.3658)
  line L529 (-8.5933, 83.3658) -> (-8.5933, 81.3658)
  line L530 (-12.5933, 81.3658) -> (-14.5933, 81.3658)
  line L531 (-14.5933, 81.3658) -> (-14.5933, 83.3658)
  line L532 (-14.5933, 83.3658) -> (-12.5933, 83.3658)
  line L533 (-12.5933, 83.3658) -> (-12.5933, 81.3658)
  line L534 (-16.5933, 81.3658) -> (-18.5933, 81.3658)
  line L535 (-18.5933, 81.3658) -> (-18.5933, 83.3658)
  line L536 (-18.5933, 83.3658) -> (-16.5933, 83.3658)
  line L537 (-16.5933, 83.3658) -> (-16.5933, 81.3658)
  line L538 (-20.5933, 81.3658) -> (-22.5933, 81.3658)
  line L539 (-22.5933, 81.3658) -> (-22.5933, 83.3658)
  line L540 (-22.5933, 83.3658) -> (-20.5933, 83.3658)
  line L541 (-20.5933, 83.3658) -> (-20.5933, 81.3658)
  line L542 (35.4067, 86.8658) -> (33.4067, 86.8658)
  line L543 (33.4067, 86.8658) -> (33.4067, 88.8658)
  line L544 (33.4067, 88.8658) -> (35.4067, 88.8658)
  line L545 (35.4067, 88.8658) -> (35.4067, 86.8658)
  line L546 (31.4067, 86.8658) -> (29.4067, 86.8658)
  line L547 (29.4067, 86.8658) -> (29.4067, 88.8658)
  line L548 (29.4067, 88.8658) -> (31.4067, 88.8658)
  line L549 (31.4067, 88.8658) -> (31.4067, 86.8658)
  line L550 (27.4067, 86.8658) -> (25.4067, 86.8658)
  line L551 (25.4067, 86.8658) -> (25.4067, 88.8658)
  line L552 (25.4067, 88.8658) -> (27.4067, 88.8658)
  line L553 (27.4067, 88.8658) -> (27.4067, 86.8658)
  line L554 (23.4067, 86.8658) -> (21.4067, 86.8658)
  line L555 (21.4067, 86.8658) -> (21.4067, 88.8658)
  line L556 (21.4067, 88.8658) -> (23.4067, 88.8658)
  line L557 (23.4067, 88.8658) -> (23.4067, 86.8658)
  line L558 (19.4067, 86.8658) -> (17.4067, 86.8658)
  line L559 (17.4067, 86.8658) -> (17.4067, 88.8658)
  line L560 (17.4067, 88.8658) -> (19.4067, 88.8658)
  line L561 (19.4067, 88.8658) -> (19.4067, 86.8658)
  line L562 (15.4067, 86.8658) -> (13.4067, 86.8658)
  line L563 (13.4067, 86.8658) -> (13.4067, 88.8658)
  line L564 (13.4067, 88.8658) -> (15.4067, 88.8658)
  line L565 (15.4067, 88.8658) -> (15.4067, 86.8658)
  line L566 (11.4067, 86.8658) -> (9.4067, 86.8658)
  line L567 (9.4067, 86.8658) -> (9.4067, 88.8658)
  line L568 (9.4067, 88.8658) -> (11.4067, 88.8658)
  line L569 (11.4067, 88.8658) -> (11.4067, 86.8658)
  line L570 (7.4067, 86.8658) -> (5.4067, 86.8658)
  line L571 (5.4067, 86.8658) -> (5.4067, 88.8658)
  line L572 (5.4067, 88.8658) -> (7.4067, 88.8658)
  line L573 (7.4067, 88.8658) -> (7.4067, 86.8658)
  line L574 (3.4067, 86.8658) -> (1.4067, 86.8658)
  line L575 (1.4067, 86.8658) -> (1.4067, 88.8658)
  line L576 (1.4067, 88.8658) -> (3.4067, 88.8658)
  line L577 (3.4067, 88.8658) -> (3.4067, 86.8658)
  line L578 (-0.5933, 86.8658) -> (-2.5933, 86.8658)
  line L579 (-2.5933, 86.8658) -> (-2.5933, 88.8658)
  line L580 (-2.5933, 88.8658) -> (-0.5933, 88.8658)
  line L581 (-0.5933, 88.8658) -> (-0.5933, 86.8658)
  line L582 (-4.5933, 86.8658) -> (-6.5933, 86.8658)
  line L583 (-6.5933, 86.8658) -> (-6.5933, 88.8658)
  line L584 (-6.5933, 88.8658) -> (-4.5933, 88.8658)
  line L585 (-4.5933, 88.8658) -> (-4.5933, 86.8658)
  line L586 (-8.5933, 86.8658) -> (-10.5933, 86.8658)
  line L587 (-10.5933, 86.8658) -> (-10.5933, 88.8658)
  line L588 (-10.5933, 88.8658) -> (-8.5933, 88.8658)
  line L589 (-8.5933, 88.8658) -> (-8.5933, 86.8658)
  line L590 (-12.5933, 86.8658) -> (-14.5933, 86.8658)
  line L591 (-14.5933, 86.8658) -> (-14.5933, 88.8658)
  line L592 (-14.5933, 88.8658) -> (-12.5933, 88.8658)
  line L593 (-12.5933, 88.8658) -> (-12.5933, 86.8658)
  line L594 (-16.5933, 86.8658) -> (-18.5933, 86.8658)
  line L595 (-18.5933, 86.8658) -> (-18.5933, 88.8658)
  line L596 (-18.5933, 88.8658) -> (-16.5933, 88.8658)
  line L597 (-16.5933, 88.8658) -> (-16.5933, 86.8658)
  line L598 (-20.5933, 86.8658) -> (-22.5933, 86.8658)
  line L599 (-22.5933, 86.8658) -> (-22.5933, 88.8658)
  line L600 (-22.5933, 88.8658) -> (-20.5933, 88.8658)
  line L601 (-20.5933, 88.8658) -> (-20.5933, 86.8658)
  line L602 (35.4067, 92.3658) -> (33.4067, 92.3658)
  line L603 (33.4067, 92.3658) -> (33.4067, 94.3658)
  line L604 (33.4067, 94.3658) -> (35.4067, 94.3658)
  line L605 (35.4067, 94.3658) -> (35.4067, 92.3658)
  line L606 (31.4067, 92.3658) -> (29.4067, 92.3658)
  line L607 (29.4067, 92.3658) -> (29.4067, 94.3658)
  line L608 (29.4067, 94.3658) -> (31.4067, 94.3658)
  line L609 (31.4067, 94.3658) -> (31.4067, 92.3658)
  line L610 (27.4067, 92.3658) -> (25.4067, 92.3658)
  line L611 (25.4067, 92.3658) -> (25.4067, 94.3658)
  line L612 (25.4067, 94.3658) -> (27.4067, 94.3658)
  line L613 (27.4067, 94.3658) -> (27.4067, 92.3658)
  line L614 (23.4067, 92.3658) -> (21.4067, 92.3658)
  line L615 (21.4067, 92.3658) -> (21.4067, 94.3658)
  line L616 (21.4067, 94.3658) -> (23.4067, 94.3658)
  line L617 (23.4067, 94.3658) -> (23.4067, 92.3658)
  line L618 (19.4067, 92.3658) -> (17.4067, 92.3658)
  line L619 (17.4067, 92.3658) -> (17.4067, 94.3658)
  line L620 (17.4067, 94.3658) -> (19.4067, 94.3658)
  line L621 (19.4067, 94.3658) -> (19.4067, 92.3658)
  line L622 (15.4067, 92.3658) -> (13.4067, 92.3658)
  line L623 (13.4067, 92.3658) -> (13.4067, 94.3658)
  line L624 (13.4067, 94.3658) -> (15.4067, 94.3658)
  line L625 (15.4067, 94.3658) -> (15.4067, 92.3658)
  line L626 (11.4067, 92.3658) -> (9.4067, 92.3658)
  line L627 (9.4067, 92.3658) -> (9.4067, 94.3658)
  line L628 (9.4067, 94.3658) -> (11.4067, 94.3658)
  line L629 (11.4067, 94.3658) -> (11.4067, 92.3658)
  line L630 (7.4067, 92.3658) -> (5.4067, 92.3658)
  line L631 (5.4067, 92.3658) -> (5.4067, 94.3658)
  line L632 (5.4067, 94.3658) -> (7.4067, 94.3658)
  line L633 (7.4067, 94.3658) -> (7.4067, 92.3658)
  line L634 (3.4067, 92.3658) -> (1.4067, 92.3658)
  line L635 (1.4067, 92.3658) -> (1.4067, 94.3658)
  line L636 (1.4067, 94.3658) -> (3.4067, 94.3658)
  line L637 (3.4067, 94.3658) -> (3.4067, 92.3658)
  line L638 (-0.5933, 92.3658) -> (-2.5933, 92.3658)
  line L639 (-2.5933, 92.3658) -> (-2.5933, 94.3658)
  line L640 (-2.5933, 94.3658) -> (-0.5933, 94.3658)
  line L641 (-0.5933, 94.3658) -> (-0.5933, 92.3658)
  line L642 (-4.5933, 92.3658) -> (-6.5933, 92.3658)
  line L643 (-6.5933, 92.3658) -> (-6.5933, 94.3658)
  line L644 (-6.5933, 94.3658) -> (-4.5933, 94.3658)
  line L645 (-4.5933, 94.3658) -> (-4.5933, 92.3658)
  line L646 (-8.5933, 92.3658) -> (-10.5933, 92.3658)
  line L647 (-10.5933, 92.3658) -> (-10.5933, 94.3658)
  line L648 (-10.5933, 94.3658) -> (-8.5933, 94.3658)
  line L649 (-8.5933, 94.3658) -> (-8.5933, 92.3658)
  line L650 (-12.5933, 92.3658) -> (-14.5933, 92.3658)
  line L651 (-14.5933, 92.3658) -> (-14.5933, 94.3658)
  line L652 (-14.5933, 94.3658) -> (-12.5933, 94.3658)
  line L653 (-12.5933, 94.3658) -> (-12.5933, 92.3658)
  line L654 (-16.5933, 92.3658) -> (-18.5933, 92.3658)
  line L655 (-18.5933, 92.3658) -> (-18.5933, 94.3658)
  line L656 (-18.5933, 94.3658) -> (-16.5933, 94.3658)
  line L657 (-16.5933, 94.3658) -> (-16.5933, 92.3658)
  line L658 (-20.5933, 92.3658) -> (-22.5933, 92.3658)
  line L659 (-22.5933, 92.3658) -> (-22.5933, 94.3658)
  line L660 (-22.5933, 94.3658) -> (-20.5933, 94.3658)
  line L661 (-20.5933, 94.3658) -> (-20.5933, 92.3658)
  line L662 (35.4067, 97.8658) -> (33.4067, 97.8658)
  line L663 (33.4067, 97.8658) -> (33.4067, 99.8658)
  line L664 (33.4067, 99.8658) -> (35.4067, 99.8658)
  line L665 (35.4067, 99.8658) -> (35.4067, 97.8658)
  line L666 (31.4067, 97.8658) -> (29.4067, 97.8658)
  line L667 (29.4067, 97.8658) -> (29.4067, 99.8658)
  line L668 (29.4067, 99.8658) -> (31.4067, 99.8658)
  line L669 (31.4067, 99.8658) -> (31.4067, 97.8658)
  line L670 (27.4067, 97.8658) -> (25.4067, 97.8658)
  line L671 (25.4067, 97.8658) -> (25.4067, 99.8658)
  line L672 (25.4067, 99.8658) -> (27.4067, 99.8658)
  line L673 (27.4067, 99.8658) -> (27.4067, 97.8658)
  line L674 (23.4067, 97.8658) -> (21.4067, 97.8658)
  line L675 (21.4067, 97.8658) -> (21.4067, 99.8658)
  line L676 (21.4067, 99.8658) -> (23.4067, 99.8658)
  line L677 (23.4067, 99.8658) -> (23.4067, 97.8658)
  line L678 (19.4067, 97.8658) -> (17.4067, 97.8658)
  line L679 (17.4067, 97.8658) -> (17.4067, 99.8658)
  line L680 (17.4067, 99.8658) -> (19.4067, 99.8658)
  line L681 (19.4067, 99.8658) -> (19.4067, 97.8658)
  line L682 (15.4067, 97.8658) -> (13.4067, 97.8658)
  line L683 (13.4067, 97.8658) -> (13.4067, 99.8658)
  line L684 (13.4067, 99.8658) -> (15.4067, 99.8658)
  line L685 (15.4067, 99.8658) -> (15.4067, 97.8658)
  line L686 (11.4067, 97.8658) -> (9.4067, 97.8658)
  line L687 (9.4067, 97.8658) -> (9.4067, 99.8658)
  line L688 (9.4067, 99.8658) -> (11.4067, 99.8658)
  line L689 (11.4067, 99.8658) -> (11.4067, 97.8658)
  line L690 (7.4067, 97.8658) -> (5.4067, 97.8658)
  line L691 (5.4067, 97.8658) -> (5.4067, 99.8658)
  line L692 (5.4067, 99.8658) -> (7.4067, 99.8658)
  line L693 (7.4067, 99.8658) -> (7.4067, 97.8658)
  line L694 (3.4067, 97.8658) -> (1.4067, 97.8658)
  line L695 (1.4067, 97.8658) -> (1.4067, 99.8658)
  line L696 (1.4067, 99.8658) -> (3.4067, 99.8658)
  line L697 (3.4067, 99.8658) -> (3.4067, 97.8658)
  line L698 (-0.5933, 97.8658) -> (-2.5933, 97.8658)
  line L699 (-2.5933, 97.8658) -> (-2.5933, 99.8658)
  line L700 (-2.5933, 99.8658) -> (-0.5933, 99.8658)
  line L701 (-0.5933, 99.8658) -> (-0.5933, 97.8658)
  line L702 (-4.5933, 97.8658) -> (-6.5933, 97.8658)
  line L703 (-6.5933, 97.8658) -> (-6.5933, 99.8658)
  line L704 (-6.5933, 99.8658) -> (-4.5933, 99.8658)
  line L705 (-4.5933, 99.8658) -> (-4.5933, 97.8658)
  line L706 (-8.5933, 97.8658) -> (-10.5933, 97.8658)
  line L707 (-10.5933, 97.8658) -> (-10.5933, 99.8658)
  line L708 (-10.5933, 99.8658) -> (-8.5933, 99.8658)
  line L709 (-8.5933, 99.8658) -> (-8.5933, 97.8658)
  line L710 (-12.5933, 97.8658) -> (-14.5933, 97.8658)
  line L711 (-14.5933, 97.8658) -> (-14.5933, 99.8658)
  line L712 (-14.5933, 99.8658) -> (-12.5933, 99.8658)
  line L713 (-12.5933, 99.8658) -> (-12.5933, 97.8658)
  line L714 (-16.5933, 97.8658) -> (-18.5933, 97.8658)
  line L715 (-18.5933, 97.8658) -> (-18.5933, 99.8658)
  line L716 (-18.5933, 99.8658) -> (-16.5933, 99.8658)
  line L717 (-16.5933, 99.8658) -> (-16.5933, 97.8658)
  line L718 (-20.5933, 97.8658) -> (-22.5933, 97.8658)
  line L719 (-22.5933, 97.8658) -> (-22.5933, 99.8658)
  line L720 (-22.5933, 99.8658) -> (-20.5933, 99.8658)
  line L721 (-20.5933, 99.8658) -> (-20.5933, 97.8658)
  arc A0 (37.4474, 72.3658) -> (11.4067, 32.3658) centre (49.3198, 36.1601) ccw
  line L722 (6.4067, 32.3658) -> (131.4067, 32.3658) projected
  line L723 (131.4067, 77.3658) -> (38.923, 77.3658) projected
  arc A1 (38.923, 77.3658) -> (7.6435, 44.7803) centre (51.3198, 34.1601) ccw projected
  point P0 (0, 0)
  point P1 (38.4067, 37.3658)
  point P2 (37.4067, 38.3658)
  point P3 (35.4067, 38.3658)
  point P4 (31.4067, 38.3658)
  point P5 (27.4067, 38.3658)
  point P6 (23.4067, 38.3658)
  point P7 (19.4067, 38.3658)
  point P8 (15.4067, 38.3658)
  point P9 (11.4067, 38.3658)
  point P10 (7.4067, 38.3658)
  point P11 (3.4067, 38.3658)
  point P12 (-0.5933, 38.3658)
  point P13 (-4.5933, 38.3658)
  point P14 (-8.5933, 38.3658)
  point P15 (-12.5933, 38.3658)
  point P16 (-16.5933, 38.3658)
  point P17 (-20.5933, 38.3658)
  point P18 (35.4067, 43.8658)
  point P19 (31.4067, 43.8658)
  point P20 (27.4067, 43.8658)
  point P21 (23.4067, 43.8658)
  point P22 (19.4067, 43.8658)
  point P23 (15.4067, 43.8658)
  point P24 (11.4067, 43.8658)
  point P25 (7.4067, 43.8658)
  point P26 (3.4067, 43.8658)
  point P27 (-0.5933, 43.8658)
  point P28 (-4.5933, 43.8658)
  point P29 (-8.5933, 43.8658)
  point P30 (-12.5933, 43.8658)
  point P31 (-16.5933, 43.8658)
  point P32 (-20.5933, 43.8658)
  point P33 (35.4067, 49.3658)
  point P34 (31.4067, 49.3658)
  point P35 (27.4067, 49.3658)
  point P36 (23.4067, 49.3658)
  point P37 (19.4067, 49.3658)
  point P38 (15.4067, 49.3658)
  point P39 (11.4067, 49.3658)
  point P40 (7.4067, 49.3658)
  point P41 (3.4067, 49.3658)
  point P42 (-0.5933, 49.3658)
  point P43 (-4.5933, 49.3658)
  point P44 (-8.5933, 49.3658)
  point P45 (-12.5933, 49.3658)
  point P46 (-16.5933, 49.3658)
  point P47 (-20.5933, 49.3658)
  point P48 (35.4067, 54.8658)
  point P49 (31.4067, 54.8658)
  point P50 (27.4067, 54.8658)
  point P51 (23.4067, 54.8658)
  point P52 (19.4067, 54.8658)
  point P53 (15.4067, 54.8658)
  point P54 (11.4067, 54.8658)
  point P55 (7.4067, 54.8658)
  point P56 (3.4067, 54.8658)
  point P57 (-0.5933, 54.8658)
  point P58 (-4.5933, 54.8658)
  point P59 (-8.5933, 54.8658)
  point P60 (-12.5933, 54.8658)
  point P61 (-16.5933, 54.8658)
  point P62 (-20.5933, 54.8658)
  point P63 (35.4067, 60.3658)
  point P64 (31.4067, 60.3658)
  point P65 (27.4067, 60.3658)
  point P66 (23.4067, 60.3658)
  point P67 (19.4067, 60.3658)
  point P68 (15.4067, 60.3658)
  point P69 (11.4067, 60.3658)
  point P70 (7.4067, 60.3658)
  point P71 (3.4067, 60.3658)
  point P72 (-0.5933, 60.3658)
  point P73 (-4.5933, 60.3658)
  point P74 (-8.5933, 60.3658)
  point P75 (-12.5933, 60.3658)
  point P76 (-16.5933, 60.3658)
  point P77 (-20.5933, 60.3658)
  point P78 (35.4067, 65.8658)
  point P79 (31.4067, 65.8658)
  point P80 (27.4067, 65.8658)
  point P81 (23.4067, 65.8658)
  point P82 (19.4067, 65.8658)
  point P83 (15.4067, 65.8658)
  point P84 (11.4067, 65.8658)
  point P85 (7.4067, 65.8658)
  point P86 (3.4067, 65.8658)
  point P87 (-0.5933, 65.8658)
  point P88 (-4.5933, 65.8658)
  point P89 (-8.5933, 65.8658)
  point P90 (-12.5933, 65.8658)
  point P91 (-16.5933, 65.8658)
  point P92 (-20.5933, 65.8658)
  point P93 (35.4067, 71.3658)
  point P94 (31.4067, 71.3658)
  point P95 (27.4067, 71.3658)
  point P96 (23.4067, 71.3658)
  point P97 (19.4067, 71.3658)
  point P98 (15.4067, 71.3658)
  point P99 (11.4067, 71.3658)
  point P100 (7.4067, 71.3658)
  point P101 (3.4067, 71.3658)
  point P102 (-0.5933, 71.3658)
  point P103 (-4.5933, 71.3658)
  point P104 (-8.5933, 71.3658)
  point P105 (-12.5933, 71.3658)
  point P106 (-16.5933, 71.3658)
  point P107 (-20.5933, 71.3658)
  point P108 (35.4067, 76.8658)
  point P109 (31.4067, 76.8658)
  point P110 (27.4067, 76.8658)
  point P111 (23.4067, 76.8658)
  point P112 (19.4067, 76.8658)
  point P113 (15.4067, 76.8658)
  point P114 (11.4067, 76.8658)
  point P115 (7.4067, 76.8658)
  point P116 (3.4067, 76.8658)
  point P117 (-0.5933, 76.8658)
  point P118 (-4.5933, 76.8658)
  point P119 (-8.5933, 76.8658)
  point P120 (-12.5933, 76.8658)
  point P121 (-16.5933, 76.8658)
  point P122 (-20.5933, 76.8658)
  point P123 (35.4067, 82.3658)
  point P124 (31.4067, 82.3658)
  point P125 (27.4067, 82.3658)
  point P126 (23.4067, 82.3658)
  point P127 (19.4067, 82.3658)
  point P128 (15.4067, 82.3658)
  point P129 (11.4067, 82.3658)
  point P130 (7.4067, 82.3658)
  point P131 (3.4067, 82.3658)
  point P132 (-0.5933, 82.3658)
  point P133 (-4.5933, 82.3658)
  point P134 (-8.5933, 82.3658)
  point P135 (-12.5933, 82.3658)
  point P136 (-16.5933, 82.3658)
  point P137 (-20.5933, 82.3658)
  point P138 (35.4067, 87.8658)
  point P139 (31.4067, 87.8658)
  point P140 (27.4067, 87.8658)
  point P141 (23.4067, 87.8658)
  point P142 (19.4067, 87.8658)
  point P143 (15.4067, 87.8658)
  point P144 (11.4067, 87.8658)
  point P145 (7.4067, 87.8658)
  point P146 (3.4067, 87.8658)
  point P147 (-0.5933, 87.8658)
  point P148 (-4.5933, 87.8658)
  point P149 (-8.5933, 87.8658)
  point P150 (-12.5933, 87.8658)
  point P151 (-16.5933, 87.8658)
  point P152 (-20.5933, 87.8658)
  point P153 (35.4067, 93.3658)
  point P154 (31.4067, 93.3658)
  point P155 (27.4067, 93.3658)
  point P156 (23.4067, 93.3658)
  point P157 (19.4067, 93.3658)
  point P158 (15.4067, 93.3658)
  point P159 (11.4067, 93.3658)
  point P160 (7.4067, 93.3658)
  point P161 (3.4067, 93.3658)
  point P162 (-0.5933, 93.3658)
  point P163 (-4.5933, 93.3658)
  point P164 (-8.5933, 93.3658)
  point P165 (-12.5933, 93.3658)
  point P166 (-16.5933, 93.3658)
  point P167 (-20.5933, 93.3658)
  point P168 (35.4067, 98.8658)
  point P169 (31.4067, 98.8658)
  point P170 (27.4067, 98.8658)
  point P171 (23.4067, 98.8658)
  point P172 (19.4067, 98.8658)
  point P173 (15.4067, 98.8658)
  point P174 (11.4067, 98.8658)
  point P175 (7.4067, 98.8658)
  point P176 (3.4067, 98.8658)
  point P177 (-0.5933, 98.8658)
  point P178 (-4.5933, 98.8658)
  point P179 (-8.5933, 98.8658)
  point P180 (-12.5933, 98.8658)
  point P181 (-16.5933, 98.8658)
  point P182 (-20.5933, 98.8658)
  point P183 (29.8922, 72.3658)
  point P184 (29.4067, 72.101)
  point P185 (10.0859, 48.3658)
  point P186 (9.5188, 46.3658)
  point P187 (27.4067, 70.9178)
  point P188 (26.5546, 70.3658)
  point P189 (23.4067, 68.0473)
  point P190 (22.5899, 67.3658)
  point P191 (21.4648, 66.3658)
  point P192 (21.4067, 66.312)
  point P193 (18.528, 63.3658)
  point P194 (17.4067, 62.0413)
  point P195 (14.1261, 57.3658)
  point P196 (13.4067, 56.1233)
  point P197 (11.1483, 51.3658)
  point P198 (10.4111, 49.3658)
  point P199 (30.6333, 69.3658)
  dimension "d90" = 2
  dimension "d91" = 2
  dimension "d92" = 0
  dimension "d93" = 2
  dimension "d96" = 4
  dimension "d99" = 5.5
  dimension "d102" = 0
  dimension "d103" = 5
  dimension "d104" = 5
  dimension "d105" = 2
  dimension "d106" = 2
  constraints: 1440 end point, 3 midpoint, 2 collinear, 2 horizontal, 2 parallel, 1 perpendicular, 1 vertical, 1613 other
  measures "d90" distance of L0.start L0.end
  measures "d91" distance of L2.end L0.start
  measures "d92" vertical distance of point (38.407, 37.366) L0.start
  measures "d93" distance of point (37.407, 38.366) point (35.407, 38.366)
  measures "d96" distance of L0.start L6.start
  measures "d99" distance of L0.start L62.start